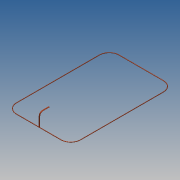
# Autodesk Inventor part: groundingPerimeter
Saved by Autodesk Inventor 2014 SP1 (Build 180222100, 222)
## iProperties
Created: 2014-12-12
Part Number: groundingPerimeter
Material: Copper
Document SubType Name: Modeling
Designer: Dave
Mass: 3467.45 g
Surface Area: 1551.43 cm^2
Volume: 387.858 cm^3
Density: 8.94 g/cm^3
Appearance: Copper - Satin
Author: Dave
Autodesk Inventor part; units mm, degrees
ref_plane "YZ Plane" through (0, 0, 0) normal (1, 0, 0) x (0, 1, 0)
ref_plane "XZ Plane" through (0, 0, 0) normal (0, 1, 0) x (-1, 0, 0)
ref_plane "XY Plane" through (0, 0, 0) normal (0, 0, 1) x (1, 0, 0)
sketch "Sketch1" plane through (0, 0, 0) normal (0, 0, 1) x (1, 0, 0)
  circle A0 centre (0, 0) radius 5
  dimension "d0" = 10
  constraints: 1 centre point, 1 coincident
  measures "d0" diameter of A0
sketch "Sketch2" plane through (0, 0, 0) normal (0, 1, 0) x (-1, 0, 0)
  line L0 (152.4, -936.5652) -> (847.6, -936.5652)
  line L1 (1000, -784.1652) -> (1000, 511.0348)
  line L2 (847.6, 663.4348) -> (152.4, 663.4348)
  line L3 (0, 511.0348) -> (0, -784.1652)
  arc A0 (152.4, 663.4348) -> (0, 511.0348) centre (152.4, 511.0348) ccw
  arc A1 (1000, 511.0348) -> (847.6, 663.4348) centre (847.6, 511.0348) ccw
  arc A2 (847.6, -936.5652) -> (1000, -784.1652) centre (847.6, -784.1652) ccw
  arc A3 (0, -784.1652) -> (152.4, -936.5652) centre (152.4, -784.1652) ccw
  point P0 (0, 0)
  point P1 (0, -936.5652)
  point P2 (1000, -936.5652)
  point P3 (0, 663.4348)
  dimension "d1" = 1600
  dimension "d2" = 1000
  dimension "d3" = 152.4
  constraints: 8 end point, 8 point on circle, 8 tangent, 6 point on line, 4 centre point, 3 equal radius, 2 parallel, 1 horizontal, 1 perpendicular
  measures "d1" distance of point (0, 663.435) point (0, -936.565)
  measures "d2" distance of point (0, -936.565) point (1000, -936.565)
  measures "d3" radius of A0
sweep "Sweep1" add profiles "Sketch1" path "Sketch2" path curves L3 A3 L0 A2 L1 A1 L2 A0
sketch "Sketch3" plane through (0, 0, 0) normal (0, 1, 0) x (-1, 0, 0)
  line L0 (480.4774, 662.2546) -> (497.6346, 662.2546)
  line L1 (497.6346, 662.2546) -> (497.6346, 665.4715)
  line L2 (497.6346, 665.4715) -> (480.4774, 665.4715)
  line L3 (480.4774, 665.4715) -> (480.4774, 662.2546)
  point P0 (0, 0)
  constraints: 8 end point, 2 parallel, 1 horizontal, 1 perpendicular
extrude "Extrusion1" add sketch "Sketch3" along normal blind 50.8
sketch "Sketch4" plane through (0, 50.8, 0) normal (0, 1, 0) x (1, 0, 0)
  line L0 (-480.4774, -662.2546) -> (-497.6346, -662.2546) projected
  line L1 (-497.6346, -662.2546) -> (-497.6346, -665.4715) projected
  line L2 (-497.6346, -665.4715) -> (-480.4774, -665.4715) projected
  line L3 (-480.4774, -665.4715) -> (-480.4774, -662.2546) projected
  point P0 (0, 0)
sketch "Sketch5" plane through (-480.4774, 4.5664, 665.4715) normal (1, 0, 0) x (0, 0, -1)
  line L0 (0, 46.2336) -> (3.217, 46.2336) projected
  line L1 (154.0085, 198.6336) -> (52.4085, 198.6336)
  line L2 (1.6085, 147.8336) -> (1.6085, 46.2336)
  arc A0 (52.4085, 198.6336) -> (1.6085, 147.8336) centre (52.4085, 147.8336) ccw
  point P0 (665.4715, -4.5664)
  point P1 (1.6085, 198.6336)
  dimension "d7" = 152.4
  dimension "d9" = 50.8
  constraints: 4 end point, 2 point on circle, 2 point on line, 2 tangent, 1 centre point, 1 midpoint
  measures "d7" distance of point (1.608, 198.634) L1.start
  measures "d9" radius of A0
sweep "Sweep2" add profiles "Sketch4" path "Sketch5" path curves L2 A0 L1
body "Solid1"
